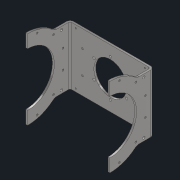
# Autodesk Inventor part: unit-plate4
Saved by Autodesk Inventor 2021 (Build 250183000, 183)
## iProperties
Created: 2021-07-14
Part Number: unit-plate4
Material: 鋼、炭素鋼
Document SubType Name: Sheet Metal
Designer: yuta0
Density: 7.85 g/cm^3
Sheet Metal Rule: Default_mm
Appearance: 半つや出し
Mass: 456.6 g
Surface Area: 415.128 cm^2
Volume: 58.1656 cm^3
Author: yuta0
Autodesk Inventor part; units mm, degrees
ref_plane "YZ Plane" through (0, 0, 0) normal (1, 0, 0) x (0, 1, 0)
ref_plane "XZ Plane" through (0, 0, 0) normal (0, 1, 0) x (-1, 0, 0)
ref_plane "XY Plane" through (0, 0, 0) normal (0, 0, 1) x (1, 0, 0)
sketch "スケッチ1" plane through (0, 0, 0) normal (0, 0, 1) x (1, 0, 0)
  line L0 (-71.7, -67.5) -> (71.7, -67.5)
  line L1 (71.7, -67.5) -> (71.7, 67.5)
  line L2 (71.7, 67.5) -> (-71.7, 67.5)
  line L3 (-71.7, 67.5) -> (-71.7, -67.5)
  line L4 (-71.7, -67.5) -> (71.7, 67.5) construction
  line L5 (71.7, -67.5) -> (-71.7, 67.5) construction
  point P0 (0, 0)
  dimension "d1" = 135
  dimension "d2" = 143.4
  measures "d1" distance of L2.end L0.start
  measures "d2" distance of L1.end L2.end
extrude "プレート1" add sketch "スケッチ1" along normal blind 3.2
sketch "スケッチ2" plane through (-68.5, -67.5, 0) normal (-1, 0, 0) x (0, -1, 0)
  line L0 (-135, 0) -> (0, 0)
  line L1 (0, 0) -> (0, 143)
  line L2 (0, 143) -> (-135, 143)
  line L3 (-135, 143) -> (-135, 0)
  constraints: 6 end point, 1 horizontal, 1 perpendicular, 1 vertical
edge flange "フランジ1" height 143 angle 90 thickness 3.2 bend radius 3.2 thickness toward (-1, 0, 0) relief tear relief width 3.2 relief depth 1.6 corner gap 3.2 corner form 0 edges at (-71.7, 0, 3.2) (71.7, 0, 3.2) wall of the first edge with corners at (-68.5, 67.5, 0) (-68.5, -67.5, 0) (-68.5, -67.5, 143) (-68.5, 67.5, 143)
bend "曲げ1"
corner "コーナー1"
sketch "スケッチ4" plane through (71.7, -67.5, 6.4) normal (1, 0, 0) x (0, 0, -1)
  circle A0 centre (-69.1, 67.5) radius 45.5
  line L0 (-136.6, 0) -> (-136.6, 135) projected
  line L1 (-136.6, 135) -> (0, 135) projected
  point P0 (6.4, 67.5)
  dimension "d17" = 91
  dimension "d54" = 67.5
  dimension "d55" = 67.5
  constraints: 1 centre point
  measures "d17" diameter of A0
  measures "d54" distance from line of L0 A0.centre
  measures "d55" distance from line of L1 A0.centre
extrude "押し出し2" cut sketch "スケッチ4" against normal through all
sketch "スケッチ5" plane through (71.7, -67.5, 6.4) normal (1, 0, 0) x (0, 0, -1)
  circle A0 centre (-69.1, 67.5) radius 62.5
  circle A1 centre (-69.1, 67.5) radius 45.5 projected
  point P0 (6.4, 67.5)
  point P1 (-129.4704, 51.3238)
  point P2 (-113.2942, 23.3058)
  point P3 (-85.2762, 7.1296)
  point P4 (-52.9238, 7.1296)
  point P5 (-24.9058, 23.3058)
  point P6 (-8.7296, 51.3238)
  point P7 (-8.7296, 83.6762)
  point P8 (-24.9058, 111.6942)
  point P9 (-52.9238, 127.8704)
  point P10 (-85.2762, 127.8704)
  point P11 (-113.2942, 111.6942)
  point P12 (-129.4704, 83.6762)
  dimension "d20" = 125
  dimension "d23" = 360
  dimension "d71" = 0
  constraints: 1 coincident, 16 other
  measures "d71" horizontal distance of point (-129.47, 83.676) point (-129.47, 51.324)
hole "穴1" at (71.7, 16.1762, 135.8704) at (71.7, 44.1942, 119.6942) at (71.7, 60.3704, 91.6762) at (71.7, 60.3704, 59.3238) at (71.7, 44.1942, 31.3058) at (71.7, -16.1762, 15.1296) at (71.7, -44.1942, 31.3058) at (71.7, -60.3704, 59.3238) at (71.7, -60.3704, 91.6762) at (71.7, -44.1942, 119.6942) at (71.7, -16.1762, 135.8704) at (71.7, 16.1762, 15.1296) direction (-1, 0, 0) diameter 3.242 end through all thread size "M4x0.7" class "6H" standard "ANSI Metric M Profile"
sketch "スケッチ6" plane through (0, 0, 3.2) normal (0, 0, 1) x (1, 0, 0)
  circle A0 centre (0, 0) radius 32
  point P0 (0, 32)
  point P1 (-27.7128, 16)
  point P2 (-27.7128, -16)
  point P3 (0, -32)
  point P4 (27.7128, -16)
  point P5 (27.7128, 16)
  dimension "d32" = 64
  dimension "d35" = 360
  constraints: 1 coincident, 1 vertical alignment, 9 other
hole "穴2" at (0, 32, 3.2) at (-27.7128, 16, 3.2) at (-27.7128, -16, 3.2) at (0, -32, 3.2) at (27.7128, -16, 3.2) at (27.7128, 16, 3.2) direction (0, 0, -1) diameter 4.3 end through all clearance for "Flat Head Machine Screw" size "M4" standard "Ansi Metric M Profile"
sketch "スケッチ7" plane through (0, 0, 3.2) normal (0, 0, 1) x (1, 0, 0)
  circle A0 centre (0, 0) radius 28
  dimension "d44" = 56
  constraints: 1 centre point, 1 coincident
  measures "d44" diameter of A0
extrude "押し出し3" cut sketch "スケッチ7" against normal blind 10
sketch "スケッチ8" plane through (71.7, -67.5, 6.4) normal (1, 0, 0) x (0, 0, -1)
  line L0 (-136.6, 0) -> (-69.1, 0)
  line L1 (-69.1, 0) -> (-69.1, 135)
  line L2 (-69.1, 135) -> (-136.6, 135)
  line L3 (-136.6, 135) -> (-136.6, 0)
  circle A0 centre (-69.1, 67.5) radius 45.5 projected
  line L4 (0, 0) -> (-136.6, 0) projected
  line L5 (-136.6, 135) -> (0, 135) projected
  point P0 (6.4, 67.5)
  dimension "d56" = 0
  constraints: 9 end point, 2 parallel, 2 point on line, 1 horizontal, 1 perpendicular
  measures "d56" distance from line of A0.centre L1
extrude "押し出し4" cut sketch "スケッチ8" against normal through all contours L3 L2 L1 A0 L0 | A0 L1 picked at (-81.4377, 82.6667)
sketch "スケッチ15" plane through (0, 0, 3.2) normal (0, 0, 1) x (1, 0, 0)
  line L0 (-47.45, -20) -> (47.45, -20)
  line L1 (47.45, -20) -> (47.45, 20)
  line L2 (47.45, 20) -> (-47.45, 20)
  line L3 (-47.45, 20) -> (-47.45, -20)
  line L4 (-47.45, -20) -> (47.45, 20) construction
  line L5 (47.45, -20) -> (-47.45, 20) construction
  point P0 (0, 0)
  dimension "d122" = 94.9
  dimension "d123" = 40
  constraints: 12 end point, 2 midpoint, 2 parallel, 1 horizontal, 1 perpendicular
  measures "d122" distance of L1.end L2.end
  measures "d123" distance of L0.end L1.end
hole "穴6" at (-47.45, 20, 3.2) at (47.45, 20, 3.2) at (47.45, -20, 3.2) at (-47.45, -20, 3.2) direction (0, 0, -1) diameter 3.242 end through all thread size "M4x0.7" class "6H" standard "ANSI Metric M Profile"
sketch "スケッチ17" plane through (0, 0, 0) normal (1, 0, 0) x (0, 1, 0)
  line L0 (-67.5, 6.4) -> (-67.5, 0) projected
  line L1 (-67.5, 6.4) -> (-67.5, 75.5) projected
  line L2 (-67.5, 0) -> (-49.5, 0)
  line L3 (-49.5, 0) -> (-49.5, 29.6088)
  line L4 (-49.5, 29.6088) -> (-67.5, 29.6088)
  line L5 (-67.5, 29.6088) -> (-67.5, 0)
  arc A0 (-45.5, 75.5) -> (45.5, 75.5) centre (0, 75.5) ccw projected
  circle A1 centre (0, 75.5) radius 67.5
  point P0 (0, 0)
  dimension "d144" = 135
  dimension "d143" = 18
  constraints: 8 end point, 2 parallel, 1 coincident, 1 horizontal, 1 perpendicular, 3 other
  measures "d143" distance of L3.end L4.end
extrude "押し出し9" cut sketch "スケッチ17" along normal through all both and the other way through all contours L1 L4 L3 L2 L0 | L1 A1 L4
mirror "ミラー2" about plane through (0, 0, 0) normal (0, 1, 0) of "押し出し9"
sketch "スケッチ9" plane through (71.7, -67.5, 6.4) normal (1, 0, 0) x (0, 0, -1)
  line L0 (0, 0) -> (0, 135) projected
  line L1 (-69.1, 22) -> (-69.1, 0) projected
  line L2 (0, 0) -> (-69.1, 0) projected
  arc A0 (-69.1, 22) -> (-69.1, 113) centre (-69.1, 67.5) ccw projected
  circle A1 centre (-69.1, 67.5) radius 67.5
  line L3 (-69.1, 135) -> (0, 135) projected
  line L4 (0, 117) -> (-23.2088, 117) projected
  point P0 (6.4, 67.5)
  point P1 (-11.4, 112)
  point P2 (-64.4, 0)
  dimension "d58" = 57.7
  dimension "d60" = 135
  dimension "d147" = 5
  constraints: 1 centre point, 1 coincident
  measures "d58" distance from line of L1 point (-11.4, 112)
  measures "d60" diameter of A1
  measures "d147" distance from line of L4 point (-11.4, 112)
hole "穴3" at (71.7, 44.5, 17.8) direction (-1, 0, 0) diameter 4.3 end through all clearance for "Flat Head Machine Screw" size "M4" standard "Ansi Metric M Profile"
sketch "スケッチ13" plane through (0, 0, 3.2) normal (0, 0, 1) x (1, 0, 0)
  line L0 (58.9, -44.5) -> (-58.9, -44.5)
  line L1 (-58.9, -44.5) -> (-58.9, 44.5)
  line L2 (-58.9, 44.5) -> (58.9, 44.5)
  line L3 (58.9, 44.5) -> (58.9, -44.5)
  line L4 (58.9, -44.5) -> (-58.9, 44.5) construction
  line L5 (-58.9, -44.5) -> (58.9, 44.5) construction
  line L6 (-65.3, -49.5) -> (65.3, -49.5) projected
  point P0 (0, 0)
  dimension "d100" = 117.8
  dimension "d148" = 5
  constraints: 12 end point, 2 midpoint, 2 parallel, 1 coincident, 1 horizontal, 1 perpendicular
  measures "d100" distance of L1.end L2.end
  measures "d148" distance between parallel lines of L6 L0
hole "穴5" at (-58.9, -44.5, 3.2) at (-58.9, 44.5, 3.2) at (58.9, 44.5, 3.2) at (58.9, -44.5, 3.2) direction (0, 0, -1) diameter 2.459 end through all thread size "M3x0.5" class "6H" standard "ANSI Metric M Profile"
fillet "コーナーR9" radius 10 4 edges at (70.1, 49.5, 29.6088) (-70.1, 49.5, 29.6088) (70.1, -49.5, 29.6088) (-70.1, -49.5, 29.6088)
mirror "ミラー3" about plane through (0, 0, 0) normal (0, 1, 0) of "穴3"
equation "\"d30\" = Thickness"
equation "\"d42\" = Thickness"
equation "\"d129\" = Thickness"
equation "\"d68\" = Thickness"
equation "\"d107\" = Thickness"
equation "\"d3\" = Thickness"
equation "\"d4\" = BendReliefWidth"
equation "\"d5\" = BendReliefDepth"
equation "\"d6\" = MinimumRemnant"
equation "\"d7\" = TransitionRadius"
equation "\"d10\" = BendRadius"
equation "\"d11\" = CornerReliefSize"
equation "\"d12\" = GapSize"
equation "\"d13\" = JacobiRadiusSize"
equation "\"BendRadius\" = Thickness"
equation "\"BendReliefWidth\" = Thickness"
equation "\"BendReliefDepth\" = 0.5 * Thickness"
equation "\"CornerReliefSize\" = 4 * Thickness"
equation "\"MinimumRemnant\" = 2 * Thickness"
equation "\"TransitionRadius\" = BendRadius"
equation "\"JacobiRadiusSize\" = BendRadius"
equation "\"GapSize\" = Thickness"
equation "\"Thickness\" = 3.2"
